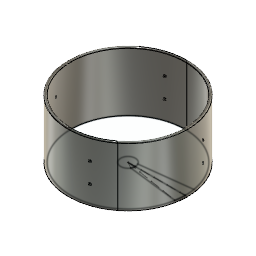
modified_drum (12) (Autodesk Fusion 360 design; units mm, degrees)
Autodesk Fusion 360 part; units mm, degrees
note: some values were not read from the file. Set by a fixed rule: which face or edge a step refers to.
sketch "Sketch1" plane through (0, 0, 0) normal (0, 0, 1) x (1, 0, 0)
  arc A0 (144.8421, 47.3977) -> (-93.659, 120.2237) centre (0, 0) ccw
  line L0 (0, 0) -> (144.8421, 47.3977) construction
  line L1 (0, 0) -> (-93.659, 120.2237) construction
  arc A1 (141.9908, 46.4646) -> (-91.8154, 117.8571) centre (0, 0) ccw
  arc A2 (139.1396, 45.5316) -> (-89.9717, 115.4905) centre (0, 0) ccw
  line L2 (-93.659, 120.2237) -> (-89.9717, 115.4905)
  line L3 (144.8421, 47.3977) -> (139.1396, 45.5316)
  arc A3 (4.468, 152.3345) -> (-93.659, 120.2237) centre (0, 0) ccw
  line L4 (0, 0) -> (4.468, 152.3345) construction
  line L5 (0, 0) -> (-93.659, 120.2237) construction
  line L6 (4.468, 152.3345) -> (4.2921, 146.3371)
  line L7 (-93.659, 120.2237) -> (-89.4056, 119.6954)
  line L8 (-93.659, 120.2237) -> (-131.3256, 120.2237) construction
  line L9 (4.2921, 146.3371) -> (1.41, 149.3933)
  arc A4 (-4.468, -152.3345) -> (144.8421, 47.3977) centre (0, 0) ccw
  arc A5 (-4.2921, -146.3371) -> (139.1396, 45.5316) centre (0, 0) ccw
  line L10 (0, 0) -> (-4.468, -152.3345) construction
  line L11 (0, 0) -> (-4.468, -152.3345) construction
  line L12 (0, 0) -> (93.659, -120.2237) construction
  line L13 (-4.468, -152.3345) -> (-1.3497, -149.3939)
  arc A6 (-4.38, -149.3358) -> (141.9908, 46.4646) centre (0, 0) ccw
  line L14 (-4.468, -152.3345) -> (-4.2921, -146.3371)
  line L15 (0, 0) -> (144.8421, 47.3977) construction
  line L16 (89.9717, -115.4905) -> (89.4539, -119.6594)
  line L17 (-4.468, -152.3345) -> (-34.8478, -174.6018) construction
  line L18 (93.659, -120.2237) -> (89.9717, -115.4905)
  line L19 (144.8421, 47.3977) -> (139.1396, 45.5316)
  arc A7 (-4.468, -152.3345) -> (93.659, -120.2237) centre (0, 0) ccw
  line L20 (93.659, -120.2237) -> (89.4056, -119.6954)
  line L21 (-4.2921, -146.3371) -> (-1.41, -149.3933)
  dimension "d1" = 152.4
  dimension "d2" = 109.8
  dimension "d5" = 39.6
  dimension "d7" = 45
  dimension "d8" = 45
  dimension "d9" = 45
  dimension "d12" = 45
  constraint coincident A0.centre L0.start
  constraint parallel L1 L2
  constraint parallel L0 L3
  constraint coincident A1.start L3
  constraint coincident A1.end L2
  constraint coincident L4 L6.end
  constraint coincident A2 L6.end
  constraint horizontal L8
  constraint coincident A1 L7.end
  constraint coincident A1 L9.end
  constraint symmetric A0.centre L3 L0.start
  constraint symmetric A0.start L3 L0.end
  constraint symmetric A0.end L3 A4.start
  constraint symmetric A0 L3 A4
  constraint symmetric A1.start L3 A6.end
  constraint symmetric A1.end L3 A6.start
  constraint symmetric A1 L3 A6
  constraint symmetric A2.start L3 A5.end
  constraint symmetric A2.end L3 A5.start
  constraint symmetric A2 L3 A5
  constraint symmetric L3 A3.start L12.end
  constraint symmetric L3 A3 A7
  constraint symmetric L3 L6.end L16.start
  constraint symmetric L3 L7.end L13.end
  constraint symmetric L3 L8.end L17.end
  constraint symmetric L3 L9.end L16.end
  constraint coincident A6 L20.end
  constraint coincident A6 L21.end
  measures "d1" radius of A0
  measures "d2" angle of L0 L1
  measures "d5" angle of L4 L5
  measures "d7" angle of L6 L9
  measures "d8" angle of L18 L20
  measures "d9" angle of L14 L21
  measures "d12" angle of L2 L7
extrude "Extrude1" add sketch "Sketch1" along normal blind 152.4 contours A0 A1 L3 L6 L19 | L3 A4 A6 L18 L19 | A0 A1 A3 L6 L7 | A1 A2 L3 L6 L19 | L3 A5 A6 L18 L19 | A6 L18 L20 | A1 L6 L9 | A6 L16 L18 | A5 A6 L16 L21 makes body 1
fillet "Fillet1" radius 3 2 edges at (146.3371, -4.2921, 152.4) (120.2237, 93.659, 152.4) on bodies 1
ref_plane "WorkPlane1" through (144.8421, 47.3977, 0) normal (0.950407, 0.311008, 0) x (-0.311008, 0.950407, 0)
sketch "Sketch2" plane through (144.8421, 47.3977, 0) normal (0.950407, 0.311008, 0) x (-0.311008, 0.950407, 0)
  line L0 (0, 149.4) -> (0, 98.6)
  line L1 (0, 98.6) -> (0, 47.8)
  line L2 (152.4, 149.4) -> (-143.3902, 149.4)
  dimension "d24" = 50.8
  dimension "d25" = 50.8
  constraint vertical L0
  constraint parallel L0 L1
  constraint coincident L0.start L2
  measures "d24" distance of L0.start L0.end
  measures "d25" distance of L0.end L1.end
hole "Hole1" at (144.8421, 47.3977, 98.6) at (144.8421, 47.3977, 47.8) direction (-0.950407, -0.311008, 0) diameter 6.35 depth 12.7 tip angle 118 bodies 1
pattern_circular "C-Pattern2" count 4 over 360 about axis through (0, 0, 149.4) along (0, 0, 1) of "Hole1"
pattern_circular "C-Pattern3" count 2 over 360 about axis through (0, 0, 149.4) along (0, 0, 1) of bodies 1 makes body 2
sketch "Sketch1 (2)" plane through (0, 0, 0) normal (0, 0, 1) x (1, 0, 0) in component "Component"
  circle A0 centre (0, 0) radius 146.4
  circle A1 centre (0, 0) radius 18.5
  line L0 (0, 0) -> (146.4, 0)
  arc A2 (144.3714, -24.2872) -> (146.4, 0) centre (0, 0) ccw
  line L1 (0, 0) -> (144.3714, -24.2872) construction
  line L2 (0, 0) -> (146.4, 0) construction
  arc A3 (16.2353, -8.8694) -> (18.5, 0) centre (0, 0) ccw
  line L3 (0, 0) -> (16.2353, -8.8694) construction
  line L4 (0, 0) -> (18.5, 0) construction
  line L5 (144.3714, -24.2872) -> (16.2353, -8.8694)
  line L6 (144.3714, 24.2872) -> (16.2353, 8.8694)
  dimension "d38" = 292.8
  dimension "d39" = 37
  dimension "d40" = 9.549
  dimension "d41" = 28.648
  constraint coincident A0.centre A1.centre
  constraint coincident A0 L0.end
  constraint horizontal L0
  constraint coincident A1 A3.end
  constraint coincident L2 A3.end
  constraint symmetric A2.start L2 L6.start
  constraint symmetric L2 A3.start L6.end
  measures "d38" diameter of A0
  measures "d39" diameter of A1
  measures "d40" angle of L1 L2
  measures "d41" angle of L3 L4
extrude "Extrude1'" add sketch "Sketch1 (2)" along normal blind 5.08 separate body contours A0 A1 L0 L6 | A0 A1 L0 A2 A3 L5 | A1 A3 makes body 3 in component "Component"
sketch "Sketch3" plane through (0, 0, 5.08) normal (0, 0, 1) x (-1, 0, 0)
  arc A0 (-144.3714, 24.2872) -> (-144.3714, -24.2872) centre (0, 0) ccw
  line L0 (-144.3714, -24.2872) -> (-16.2353, -8.8694)
  arc A1 (-16.2353, -8.8694) -> (-16.2353, 8.8694) centre (0, 0) ccw
  line L1 (-16.2353, 8.8694) -> (-144.3714, 24.2872)
  circle A2 centre (0, 0) radius 18.5
  circle A3 centre (0, 0) radius 146.4
  circle A4 centre (0, 0) radius 141.32
  dimension "d44" = -5.08
extrude "Extrude2" add sketch "Sketch3" along normal blind 63.5 contours A0 L0 L1 A3 A4 bodies 3 in component "Component"
fillet "Fillet1'" offset 102.4 second offset 63.5 1 edges at (141.32, 0, 5.08) measured on face at (57.856, 2.6422, 5.08) on bodies 3 in component "Component"
shell "Shell1" thickness 2.54 removed faces 2 at (23.7969, 0, 5.08) at (97.135, -9.7925, 16.5522) on bodies 3 in component "Component"
sketch "Sketch4" plane through (0, 0, 2.54) normal (0, 0, 1) x (-1, 0, 0)
  arc A0 (-142.2483, 21.4734) -> (-142.2483, -21.4734) centre (0, 0) ccw
  line L0 (-142.2483, -21.4734) -> (-14.7356, -6.1306)
  arc A1 (-14.7356, -6.1306) -> (-14.7356, 6.1306) centre (0, 0) ccw
  line L1 (-14.7356, 6.1306) -> (-142.2483, 21.4734)
  circle A2 centre (0, 0) radius 18.5
  circle A3 centre (0, 0) radius 15.96
  dimension "d51" = -2.54
extrude "Extrude3" add sketch "Sketch4" along normal blind 6.35 contours A1 A3 bodies 3 in component "Component"
fillet "Fillet2" radius 3.81 1 edges at (-15.96, 0, 5.08) on bodies 3 in component "Component"
ref_plane "WorkPlane2" through (146.4, 0, 34.29) normal (1, 0, 0) x (0, 1, 0)
sketch "Sketch5" plane through (146.4, 0, 0) normal (1, 0, 0) x (0, 1, 0)
  line L0 (0, 68.58) -> (0, 62.23)
  line L1 (0, 62.23) -> (0, 11.43)
  line L2 (0, 11.43) -> (0, 5.08)
  circle A0 centre (0, 8.255) radius 3.175
  circle A1 centre (0, 59.055) radius 3.175
  line L3 (0, 8.255) -> (-3.175, 8.255)
  line L4 (0, 8.255) -> (3.175, 8.255)
  line L5 (0, 59.055) -> (3.175, 59.055)
  line L6 (0, 59.055) -> (-3.175, 59.055)
  line L7 (3.175, 59.055) -> (3.175, 8.255)
  line L8 (-3.175, 8.255) -> (-3.175, 59.055)
  dimension "d57" = 6.35
  dimension "d58" = 50.8
  dimension "d59" = 6.35
  dimension "d60" = 6.35
  constraint vertical L0
  constraint parallel L0 L1
  constraint parallel L1 L2
  constraint coincident L2.end A0
  constraint coincident L1.end A0
  constraint coincident L0.end A1
  constraint coincident A0.centre L3.start
  constraint coincident A0 L3.end
  constraint perpendicular L2 L3
  constraint coincident A0 L4.end
  constraint perpendicular L2 L4
  constraint coincident A1.centre L5.start
  constraint coincident A1 L5.end
  constraint perpendicular L1 L5
  constraint coincident A1 L6.end
  constraint perpendicular L1 L6
  constraint tangent A0 L7
  constraint tangent A1 L8
  measures "d57" distance of L0.start L0.end
  measures "d58" distance of L0.end L1.end
  measures "d59" distance of L1.end L2.end
  measures "d60" diameter of A1
extrude "Extrude4" cut sketch "Sketch5" against normal blind 5.08 bodies 3 in component "Component"
fillet "Fillet3" radius 5.08 tangency weight 0.81964 1 edges at (141.32, 0, 68.58) on bodies 3 in component "Component"
component "Component" placed x (1, 0, 0) y (0, 1, 0) z (0, 0, 1) at (0, 0, 0)
equation "d1 = ShellDiam / 2"
equation "d2 = PieceSize * LapSize + PieceSize"
equation "d3 = -HalfShellThick"
equation "d4 = -ShellThick"
equation "d5 = PieceSize * ( LapSize * 2 )"
equation "d10 = ShellHeight"
equation "NumSegments = 2"
equation "ShellThick = 6 mm"
equation "ShellHeight = 6 in"
equation "ShellDiam = 12 in"
equation "LapSize = LapSizePercent / 100"
equation "PieceSize = ( 180 / NumSegments ) * 1 deg"
equation "d22 = HalfShellThick"
equation "d24 = LugTopDist"
equation "d25 = LugSpacing"
equation "d27 = LugHoleDiam"
equation "d29 = NumSegments * 2"
equation "d31 = NumSegments"
equation "LugTopDist = 2 in"
equation "LugSpacing = 2 in"
equation "LapSizePercent = 22"
equation "HalfShellThick = ShellThick / 2"
equation "LugHoleDiam = 0.25 in"
equation "d38 = ShellDiam - ( ShellThick * 2 )"
equation "d40 = ( ( 360 * 1 in ) / ( PI * ShellDiam ) ) * 1 deg"
equation "d41 = ( ( 360 * 3 in ) / ( PI * ShellDiam ) ) * 1 deg"
equation "d45 = LugSpacing + ( LugHoleDiam * 2 )"
equation "d48 = ShellDiam / 2 - 50 mm"
equation "d49 = LugSpacing + ( LugHoleDiam * 2 )"
equation "d57 = LugHoleDiam"
equation "d58 = LugSpacing"
equation "d59 = LugHoleDiam"
equation "d60 = LugHoleDiam"
